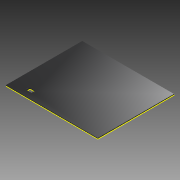
# Autodesk Inventor part: EnclosurePanelBack
Saved by Autodesk Inventor 2015 SP1 (Build 190203100, 203)
## iProperties
Category: Panel
Created: 2015-01-12
Part Number: EnclosurePanelBack
Material: ABS Plastic
Document SubType Name: Modeling
Designer: Jack
Density: 1.06 g/cm^3
Appearance: Smooth - Dark Gray
Mass: 717.302 g
Surface Area: 3450.7 cm^2
Volume: 676.7 cm^3
Vendor: Tap Plastics
Author: Jack
Autodesk Inventor part; units mm, degrees
ref_plane "YZ Plane" through (0, 0, 0) normal (1, 0, 0) x (0, 1, 0)
ref_plane "XZ Plane" through (0, 0, 0) normal (0, 1, 0) x (-1, 0, 0)
ref_plane "XY Plane" through (0, 0, 0) normal (0, 0, 1) x (1, 0, 0)
sketch "Sketch1" plane through (0, 0, 0) normal (0, 0, 1) x (1, 0, 0)
  line L0 (0, 0) -> (505, 0)
  line L1 (505, 0) -> (505, 420)
  line L2 (505, 420) -> (0, 420)
  line L3 (0, 420) -> (0, 0)
  dimension "d0" = 505
  dimension "d1" = 420
  constraints: 8 end point, 2 parallel, 1 horizontal, 1 perpendicular
  measures "d0" distance of L2.end L1.end
  measures "d1" distance of L0.end L1.end
extrude "Extrusion1" add sketch "Sketch1" along normal blind 4.7625
sketch "Sketch2" plane through (0, 0, 0) normal (0, 0, -1) x (-1, 0, 0)
  line L0 (0, 0) -> (-505, 0) projected
  line L1 (0, 420) -> (0, 0) projected
  line L2 (-107, 33) -> (-80, 33)
  line L3 (-80, 33) -> (-80, 52)
  line L4 (-80, 52) -> (-107, 52)
  line L5 (-107, 52) -> (-107, 33)
  dimension "d4" = 27
  dimension "d5" = 19
  dimension "d6" = 33
  dimension "d7" = 80
  constraints: 8 end point, 2 parallel, 1 horizontal, 1 perpendicular
  measures "d4" distance of L4.end L3.end
  measures "d5" distance of L3.end L2.end
  measures "d6" distance between parallel lines of L0 L2
  measures "d7" distance between parallel lines of L1 L3
extrude "Extrusion2" cut sketch "Sketch2" against normal up to next
sketch "Sketch3" plane through (0, 0, 0) normal (0, 0, -1) x (-1, 0, 0)
  line L0 (-80, 52) -> (-80, 33) projected
  line L1 (-107, 52) -> (-80, 52) projected
  circle A0 centre (-113.5, 42.5) radius 1.75
  circle A1 centre (-73.5, 42.5) radius 1.75
  dimension "d10" = 3.5
  dimension "d11" = 40
  dimension "d12" = 6.5
  dimension "d13" = 9.5
  constraints: 2 centre point, 1 equal radius, 1 horizontal alignment
  measures "d10" diameter of A0
  measures "d11" distance of A0.centre A1.centre
  measures "d12" distance from line of L0 A1.centre
  measures "d13" distance from line of L1 A0.centre
extrude "Extrusion3" cut sketch "Sketch3" against normal up to next
sketch "Sketch4" plane through (0, 0, 0) normal (0, 0, -1) x (-1, 0, 0)
  line L0 (0, 0) -> (-505, 0) projected
  line L1 (0, 420) -> (0, 0) projected
  line L2 (-505, 420) -> (0, 420) projected
  line L3 (-505, 0) -> (-505, 420) projected
  circle A0 centre (-495, 410) radius 2.25
  circle A1 centre (-10, 410) radius 2.25
  circle A2 centre (-10, 10) radius 2.25
  circle A3 centre (-495, 10) radius 2.25
  circle A4 centre (-252.5, 410) radius 2.25
  circle A5 centre (-252.5, 10) radius 2.25
  circle A6 centre (-10, 210) radius 2.25
  circle A7 centre (-495, 210) radius 2.25
  circle A8 centre (-252.5, 75) radius 2.25
  dimension "d16" = 10
  dimension "d17" = 4.5
  dimension "d18" = 10
  dimension "d19" = 10
  dimension "d20" = 10
  dimension "d21" = 210
  dimension "d22" = 252.5
  dimension "d23" = 75
  constraints: 9 centre point, 8 equal radius, 6 vertical alignment, 5 horizontal alignment
  measures "d16" distance from line of L0 A3.centre
  measures "d17" diameter of A3
  measures "d18" distance from line of L3 A3.centre
  measures "d19" distance from line of L2 A0.centre
  measures "d20" distance from line of L1 A2.centre
  measures "d21" distance from line of L0 A7.centre
  measures "d22" distance from line of L1 A5.centre
  measures "d23" distance from line of L0 A8.centre
extrude "Extrusion4" cut sketch "Sketch4" against normal up to next contours A0 | A1 | A2 | A3 | A4 | A5 | A6 | A7 | A8
chamfer "Chamfer1" distance 2 angle 45 9 edges at (497.25, 410, 0) (254.75, 410, 0) (12.25, 410, 0) (12.25, 210, 0) (254.75, 75, 0) (254.75, 10, 0) (12.25, 10, 0) (497.25, 10, 0) (497.25, 210, 0)
body "Solid1"
